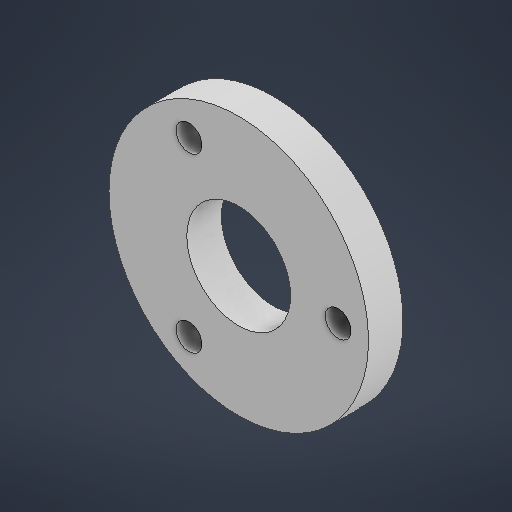
# Autodesk Inventor part: 01-03-01-02 Zeichnung Zange links oben
Saved by Autodesk Inventor 2026.2 (Build 302298000, 298)
## iProperties
Created: 2026-01-31
Part Number: 01-03-01-02 Zeichnung Zange links oben
Material: Generisch
Document SubType Name: Modeling
Designer: Schally
Density: 1 g/cm^3
Appearance: Vorgabe
Author: Schally
Autodesk Inventor part; units mm, degrees
ref_plane "YZ Plane" through (0, 0, 0) normal (1, 0, 0) x (0, 1, 0)
ref_plane "XZ Plane" through (0, 0, 0) normal (0, 1, 0) x (-1, 0, 0)
ref_plane "XY Plane" through (0, 0, 0) normal (0, 0, 1) x (1, 0, 0)
sketch "Skizze1" plane through (0, 0, 0) normal (0, 1, 0) x (-1, 0, 0)
  circle A0 centre (0, 0) radius 15
  circle A1 centre (0, 0) radius 6
  circle A2 centre (0, 0) radius 11.5
  line L0 (0, 0) -> (-26.7883, 0)
  line L1 (0, 0) -> (13.3942, -23.1994)
  line L2 (0, 0) -> (13.3942, 23.1994)
  circle A3 centre (5.75, -9.9593) radius 1.5
  circle A4 centre (5.75, 9.9593) radius 1.5
  circle A5 centre (-11.5, 0) radius 1.5
  dimension "d0" = 30
  dimension "d1" = 12
  dimension "d3" = 23
  dimension "d6" = 360
  dimension "d8" = 3
  dimension "d9" = 3
  dimension "d10" = 3
  constraints: 6 centre point, 6 end point, 3 coincident, 3 point on circle, 3 point on line, 1 horizontal, 10 other
  measures "d0" diameter of A0
  measures "d1" diameter of A1
  measures "d3" diameter of A2
  measures "d8" diameter of A3
  measures "d9" diameter of A4
  measures "d10" diameter of A5
extrude "Extrusion1" add sketch "Skizze1" along normal blind 4 contours A0 L1 A3 A2 A4 L2 | L2 A4 A2 A5 L0 A0 | A0 L0 A5 A2 A3 L1 | A4 L2 A1 L0 A5 A2 | A2 A5 L0 A1 L1 A3 | A2 A3 L1 A1 L2 A4
